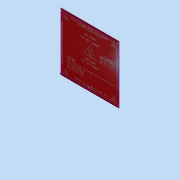
# Autodesk Inventor part: 200x200 RepRap Heated Bed
Saved by Autodesk Inventor 2015 (Build 190159000, 159)
## iProperties
Created: 2016-06-24
Part Number: 200x200 RepRap Heated Bed
Material: Generic
Document SubType Name: Modeling
Designer: Dustin
Density: 1 g/cm^3
Appearance: Default
Author: Dustin
Autodesk Inventor part; units mm, degrees
ref_plane "YZ Plane" through (0, 0, 0) normal (1, 0, 0) x (0, 1, 0)
ref_plane "XZ Plane" through (0, 0, 0) normal (0, 1, 0) x (-1, 0, 0)
ref_plane "XY Plane" through (0, 0, 0) normal (0, 0, 1) x (1, 0, 0)
sketch "Sketch3" plane through (0, 0, 0) normal (0, 0, 1) x (1, 0, 0)
  line L0 (0, 0) -> (214, 0)
  line L1 (214, 0) -> (214, 214)
  line L2 (214, 214) -> (0, 214)
  line L3 (0, 214) -> (0, 0)
  dimension "d2" = 214
  dimension "d3" = 214
  constraints: 8 end point, 2 parallel, 1 horizontal, 1 perpendicular
  measures "d2" distance of L0.start L0.end
  measures "d3" distance of L2.end L0.start
extrude "Extrusion1" add sketch "Sketch3" along normal blind 1.65
sketch "Sketch4" plane through (0, 0, 1.65) normal (0, 0, 1) x (1, 0, 0)
  line L0 (0.5008, 209.7083) -> (213.5162, 209.7083)
  line L1 (213.5162, 209.7083) -> (213.5162, 5.2135)
  line L2 (213.5162, 5.2135) -> (0.5008, 5.2135)
  line L3 (0.5008, 5.2135) -> (0.5008, 209.7083)
  constraints: 1 coincident, 2 other
sketch "Sketch5" plane through (0, 0, 1.65) normal (0, 0, 1) x (1, 0, 0)
  line L0 (214, 214) -> (0, 214) projected
  line L1 (0, 214) -> (0, 0) projected
  line L2 (214, 0) -> (214, 214) projected
  line L3 (0, 0) -> (214, 0) projected
  point P0 (3, 3)
  point P1 (211, 3)
  point P2 (211, 211)
  point P3 (3, 211)
  dimension "d41" = 3
  dimension "d42" = 3
  dimension "d43" = 3
  dimension "d44" = 3
  dimension "d45" = 3
  dimension "d46" = 3
  dimension "d47" = 3
  dimension "d48" = 3
  measures "d41" distance from line of L0 point (3, 211)
  measures "d42" distance from line of L1 point (3, 211)
  measures "d43" distance from line of L0 point (211, 211)
  measures "d44" distance from line of L2 point (211, 211)
  measures "d45" distance from line of L2 point (211, 3)
  measures "d46" distance from line of L3 point (211, 3)
  measures "d47" distance from line of L1 point (3, 3)
  measures "d48" distance from line of L3 point (3, 3)
hole "Hole1" at (3, 211, 1.65) at (3, 3, 1.65) at (211, 3, 1.65) at (211, 211, 1.65) direction (0, 0, -1) diameter 3 depth 25.4 tip angle 118
body "Solid1"
